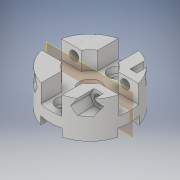
# Autodesk Inventor part: BRImp_Mount
Saved by Autodesk Inventor 2018 (Build 220112000, 112)
## iProperties
Created: 2018-02-04
Part Number: BRImp_Mount
Material: Generic
Document SubType Name: Modeling
Designer: Benedikt
Density: 1 g/cm^3
Appearance: Default
Author: Benedikt
## iProperties of the stored document BRImp_Mount_3DPrint.ipt
Created: 2018-02-04
Part Number: BRImp_Mount_3DPrint
Material: Generic
Document SubType Name: Modeling
Designer: Benedikt
Density: 1 g/cm^3
Appearance: Default
Author: Benedikt
Autodesk Inventor part; units mm, degrees
ref_plane "YZ Plane" through (0, 0, 0) normal (1, 0, 0) x (0, 1, 0)
sketch "Sketch1" plane through (0, 0, 0) normal (0, 0, 1) x (1, 0, 0)
  line L0 (-16.6854, -3.75) -> (16.6854, -3.75)
  line L1 (16.6854, -3.75) -> (16.6854, 3.75)
  line L2 (16.6854, 3.75) -> (-16.6854, 3.75)
  line L3 (-16.6854, 3.75) -> (-16.6854, -3.75)
  line L4 (-16.6854, -3.75) -> (16.6854, 3.75) construction
  line L5 (16.6854, -3.75) -> (-16.6854, 3.75) construction
  line L6 (-4, -17.2757) -> (4, -17.2757)
  line L7 (4, -17.2757) -> (4, 17.2757)
  line L8 (4, 17.2757) -> (-4, 17.2757)
  line L9 (-4, 17.2757) -> (-4, -17.2757)
  line L10 (-4, -17.2757) -> (4, 17.2757) construction
  line L11 (4, -17.2757) -> (-4, 17.2757) construction
  dimension "d4" = 7.5
  dimension "d5" = 8
  constraints: 24 end point, 4 parallel, 2 horizontal, 2 perpendicular
  measures "d4" distance of L1.end L0.end
  measures "d5" distance of L8.end L7.end
sketch "Sketch2" plane through (0, 0, 0) normal (0, 0, 1) x (1, 0, 0)
  circle A0 centre (0, 0) radius 15.3
  dimension "d6" = 30.6
  constraints: 1 centre point, 1 coincident
  measures "d6" diameter of A0
extrude "Extrusion1" add sketch "Sketch2" against normal blind 14
extrude "Extrusion2" cut sketch "Sketch1" against normal blind 7
ref_plane "Work Plane1" through (0, 15.3, 0) normal (0, 1, 0) x (-1, 0, 0)
sketch "Sketch3" plane through (0, 15.3, 0) normal (0, 1, 0) x (-1, 0, 0)
  circle A0 centre (-9.8, -2.8) radius 1.75
  line L0 (0, 4.1313) -> (0, -18.5178) construction
  circle A1 centre (9.8, -3.15) radius 1.75
  line L1 (-14.8333, 0) -> (-4, 0) projected
  line L2 (4, 0) -> (14.8333, 0) projected
  point P0 (0, 0)
  dimension "d11" = 3.5
  dimension "d12" = 9.8
  dimension "d50" = 2.8
  dimension "d53" = 3.15
  constraints: 2 centre point, 2 end point, 1 vertical
  measures "d11" diameter of A0
  measures "d12" distance from line of A0.centre L0
  measures "d50" distance from line of L1 A0.centre
  measures "d53" distance from line of L2 A1.centre
extrude "Extrusion3" cut sketch "Sketch3" against normal through all
sketch "Sketch4" plane through (0, 15.3, 0) normal (0, 1, 0) x (-1, 0, 0)
  spline S0 degree 5 poles (-8.05, -2.8) (-8.05, -2.4902) (-8.1185, -2.1805) (-8.2558, -1.8875) (-8.4573, -1.6351) (-8.8623, -1.3077) (-9.0435, -1.2017) (-9.2354, -1.125) (-9.4313, -1.0782) (-9.9507, -1.0261) (-10.2698, -1.0709) (-10.5635, -1.1818) (-10.8246, -1.3477) (-11.2231, -1.75) (-11.3733, -1.9682) (-11.4896, -2.2224) (-11.5494, -2.5096) (-11.5506, -3.0815) (-11.4926, -3.3675) (-11.3785, -3.6216) (-11.2304, -3.8399) (-10.8808, -4.1981) (-10.6823, -4.3402) (-10.4616, -4.4473) (-10.2238, -4.5163) (-9.719, -4.5669) (-9.4519, -4.5464) (-9.1808, -4.4734) (-8.9252, -4.3421) (-8.4599, -3.9681) (-8.2567, -3.7145) (-8.1192, -3.4222) (-8.05, -3.1106) (-8.05, -2.8) knots 0 0 0 0 0 0 0.134348 0.134348 0.134348 0.134348 0.224335 0.224335 0.224335 0.224335 0.375238 0.375238 0.375238 0.375238 0.499498 0.499498 0.499498 0.499498 0.623116 0.623116 0.623116 0.623116 0.742536 0.742536 0.742536 0.742536 0.865073 0.865073 0.865073 0.865073 1 1 1 1 1 1 projected
  circle A0 centre (-9.8, -2.8) radius 3.1
  circle A1 centre (-9.8, -2.8) radius 1.75 projected
  line L0 (0.004, 5.0066) -> (0.004, -21.3653) construction
  circle A2 centre (9.8, -3.15) radius 3.1
  circle A3 centre (9.8, -3.15) radius 1.75 projected
  point P0 (0, 0)
  dimension "d15" = 6.2
  constraints: 2 centre point, 2 end point, 1 concentric, 1 horizontal alignment, 1 vertical, 2 other
  measures "d15" diameter of A0
extrude "Extrusion4" cut sketch "Sketch4" against normal blind 8.45 contours A0 | A2 | A3
ref_plane "Work Plane2" through (0, -15.3, 0) normal (0, 1, 0) x (-1, 0, 0)
sketch "Sketch5" plane through (0, -15.3, 0) normal (0, 1, 0) x (-1, 0, 0)
  spline S0 degree 5 poles (11.55, -3.15) (11.55, -2.9869) (11.531, -2.8248) (11.4935, -2.6675) (11.4392, -2.5185) (11.3216, -2.2779) (11.2637, -2.1809) (11.199, -2.09) (11.1284, -2.0056) (10.8808, -1.7519) (10.6823, -1.6098) (10.4616, -1.5027) (10.2238, -1.4337) (9.719, -1.3831) (9.4519, -1.4036) (9.1808, -1.4766) (8.9252, -1.6079) (8.4606, -1.9813) (8.2581, -2.2334) (8.12, -2.5264) (8.0507, -2.8361) (8.0496, -3.3622) (8.0823, -3.5781) (8.1486, -3.788) (8.2469, -3.9854) (8.5502, -4.4125) (8.7819, -4.6241) (9.0567, -4.7767) (9.3427, -4.8629) (9.9507, -4.9239) (10.2698, -4.8791) (10.5635, -4.7682) (10.8246, -4.6023) (11.1206, -4.3035) (11.1927, -4.2185) (11.2587, -4.1268) (11.3178, -4.0288) (11.4375, -3.7863) (11.4925, -3.6363) (11.5307, -3.4778) (11.55, -3.3144) (11.55, -3.15) knots 0 0 0 0 0 0 0.070413 0.070413 0.070413 0.070413 0.123138 0.123138 0.123138 0.123138 0.242556 0.242556 0.242556 0.242556 0.36509 0.36509 0.36509 0.36509 0.499606 0.499606 0.499606 0.499606 0.593209 0.593209 0.593209 0.593209 0.724405 0.724405 0.724405 0.724405 0.875455 0.875455 0.875455 0.875455 0.928962 0.928962 0.928962 0.928962 1 1 1 1 1 1 projected
  spline S1 degree 5 poles (-8.05, -2.8) (-8.05, -2.4902) (-8.1185, -2.1805) (-8.2558, -1.8875) (-8.4573, -1.6351) (-8.8623, -1.3077) (-9.0435, -1.2017) (-9.2354, -1.125) (-9.4313, -1.0782) (-9.9507, -1.0261) (-10.2698, -1.0709) (-10.5635, -1.1818) (-10.8246, -1.3477) (-11.2231, -1.75) (-11.3733, -1.9682) (-11.4896, -2.2224) (-11.5494, -2.5096) (-11.5506, -3.0815) (-11.4926, -3.3675) (-11.3785, -3.6216) (-11.2304, -3.8399) (-10.8808, -4.1981) (-10.6823, -4.3402) (-10.4616, -4.4473) (-10.2238, -4.5163) (-9.719, -4.5669) (-9.4519, -4.5464) (-9.1808, -4.4734) (-8.9252, -4.3421) (-8.4599, -3.9681) (-8.2567, -3.7145) (-8.1192, -3.4222) (-8.05, -3.1106) (-8.05, -2.8) knots 0 0 0 0 0 0 0.134348 0.134348 0.134348 0.134348 0.224335 0.224335 0.224335 0.224335 0.375238 0.375238 0.375238 0.375238 0.499498 0.499498 0.499498 0.499498 0.623116 0.623116 0.623116 0.623116 0.742536 0.742536 0.742536 0.742536 0.865073 0.865073 0.865073 0.865073 1 1 1 1 1 1 projected
  circle A0 centre (9.8, -3.15) radius 1.75 projected
  line L0 (8.0644, -0.1521) -> (11.5285, -0.1479)
  line L1 (11.5285, -0.1479) -> (13.2641, -3.1459)
  line L2 (13.2641, -3.1459) -> (11.5356, -6.1479)
  line L3 (11.5356, -6.1479) -> (8.0715, -6.1521)
  line L4 (8.0715, -6.1521) -> (6.3359, -3.1541)
  line L5 (6.3359, -3.1541) -> (8.0644, -0.1521)
  line L6 (-151.9098, 3.5661) -> (-151.9098, -9.718) construction
  circle A1 centre (-313.6196, -3.15) radius 1.75
  line L7 (-311.884, -0.1521) -> (-315.3481, -0.1479)
  line L8 (-315.3481, -0.1479) -> (-317.0837, -3.1459)
  line L9 (-317.0837, -3.1459) -> (-315.3553, -6.1479)
  line L10 (-315.3553, -6.1479) -> (-311.8912, -6.1521)
  line L11 (-311.8912, -6.1521) -> (-310.1555, -3.1541)
  line L12 (-310.1555, -3.1541) -> (-311.884, -0.1521)
  line L13 (4, -7) -> (4, 0) projected
  line L14 (-4, 0) -> (-4, -7) projected
  line L15 (-11.458, 0.106) -> (-8.1094, 0.0939)
  line L16 (-8.1094, 0.0939) -> (-6.4456, -2.8121)
  line L17 (-6.4456, -2.8121) -> (-8.1303, -5.706)
  line L18 (-8.1303, -5.706) -> (-11.4789, -5.6939)
  line L19 (-11.4789, -5.6939) -> (-13.1428, -2.7879)
  line L20 (-13.1428, -2.7879) -> (-11.458, 0.106)
  point P0 (0, 0)
  point P1 (-315.3696, -3.15)
  point P2 (-9.7942, -2.8)
  dimension "d18" = 6
  dimension "d54" = 5.8
  constraints: 38 end point, 9 symmetric about line, 2 coincident, 2 horizontal alignment, 2 vertical, 29 other
  measures "d18" distance between parallel lines of L3 L0
  measures "d54" distance between parallel lines of L18 L15
extrude "Extrusion5" cut sketch "Sketch5" along normal blind 8.8 contours L0 L1 L2 L3 L4 L5 | A1 | L12 L11 L10 L9 L8 L7 | L15 L16 L17 L18 L19 L20
sketch "Sketch6" plane through (0, 0, -7) normal (0, 0, 1) x (1, 0, 0)
  circle A0 centre (0, 0) radius 4.1
  dimension "d21" = 8.2
  constraints: 1 centre point, 1 coincident
  measures "d21" diameter of A0
extrude "Extrusion6" cut sketch "Sketch6" against normal through all
sketch "Sketch7" plane through (0, 0, -14) normal (0, 0, -1) x (-1, 0, 0)
  circle A0 centre (0, 0) radius 4.1 projected
  circle A1 centre (0, 0) radius 15.3 projected
  circle A2 centre (0, 0) radius 7.5
  circle A3 centre (0, 0) radius 12.5
  line L0 (-50, 4) -> (50, 4)
  line L1 (50, 4) -> (50, -4)
  line L2 (50, -4) -> (-50, -4)
  line L3 (-50, -4) -> (-50, 4)
  line L4 (-50, 4) -> (50, -4) construction
  line L5 (50, 4) -> (-50, -4) construction
  line L6 (4, 50) -> (-4, 50)
  line L7 (-4, 50) -> (-4, -50)
  line L8 (-4, -50) -> (4, -50)
  line L9 (4, -50) -> (4, 50)
  line L10 (4, 50) -> (-4, -50) construction
  line L11 (-4, 50) -> (4, -50) construction
  dimension "d24" = 15
  dimension "d25" = 25
  dimension "d28" = 100
  dimension "d29" = 8
  dimension "d30" = 8
  dimension "d31" = 100
  constraints: 24 end point, 4 midpoint, 4 parallel, 2 centre point, 2 coincident, 2 horizontal, 2 perpendicular
  measures "d24" diameter of A2
  measures "d25" diameter of A3
  measures "d28" distance of L1.end L2.end
  measures "d29" distance between parallel lines of L0 L2
  measures "d30" distance of L8.end L7.end
  measures "d31" distance of L7.end L6.end
extrude "Extrusion7" cut sketch "Sketch7" against normal blind 3 contours L0 A3 L2 A2 | A2 L9 A3 L0 | A2 L7 A3 L9 | L2 A3 L9 A2 | L9 A3 L7 A2 | A2 L0 A3 L7 | L7 A3 L2 A2 | A2 L2 A3 L0
sketch "Sketch8" plane through (0, 0, -14) normal (0, 0, -1) x (-1, 0, 0)
  line L0 (4.1, 18.3809) -> (-4.1, 18.3809)
  line L1 (-4.1, 18.3809) -> (-4.1, -18.3809)
  line L2 (-4.1, -18.3809) -> (4.1, -18.3809)
  line L3 (4.1, -18.3809) -> (4.1, 18.3809)
  line L4 (4.1, 18.3809) -> (-4.1, -18.3809) construction
  line L5 (-4.1, 18.3809) -> (4.1, -18.3809) construction
  line L6 (19.6063, -4.1) -> (-19.6063, -4.1)
  line L7 (-19.6063, -4.1) -> (-19.6063, 4.1)
  line L8 (-19.6063, 4.1) -> (19.6063, 4.1)
  line L9 (19.6063, 4.1) -> (19.6063, -4.1)
  line L10 (19.6063, -4.1) -> (-19.6063, 4.1) construction
  line L11 (-19.6063, -4.1) -> (19.6063, 4.1) construction
  circle A0 centre (0, 0) radius 8.9501
  dimension "d32" = 8.2
  dimension "d33" = 8.2
  constraints: 24 end point, 4 midpoint, 4 parallel, 2 horizontal, 2 perpendicular, 1 centre point, 1 coincident
  measures "d32" distance of L2.end L1.end
  measures "d33" distance of L6.end L7.end
extrude "Extrusion8" cut sketch "Sketch8" against normal blind 3
sketch "Sketch9" plane through (0, 0, -7) normal (0, 0, 1) x (1, 0, 0)
  point P0 (0, 0)
  point P1 (0, -10)
  dimension "d39" = 10
  measures "d39" distance of point (0, 0) point (0, -10)
hole "Hole1" at (0, -10, -7) direction (0, 0, -1) diameter 3.4 depth 8 tip angle 118 counterbore diameter 6 counterbore depth 2.5
ref_plane "Work Plane3" through (-14.8333, 0, -7) normal (0, -1, 0) x (1, 0, 0)
mirror "Mirror1" about plane through (-14.8333, 0, -7) normal (0, -1, 0) of "Hole1"
sketch "Sketch10" plane through (0, 0, 0) normal (0, 0, 1) x (1, 0, 0)
  circle A0 centre (0, 0) radius 8
  dimension "d47" = 16
  constraints: 1 centre point, 1 coincident
  measures "d47" diameter of A0
extrude "Extrusion9" cut sketch "Sketch10" against normal up to surface (7 mm away)
body "Solid1"
